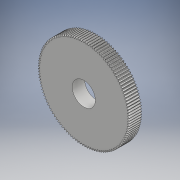
# Autodesk Inventor part: Колесо 1
Saved by Autodesk Inventor 2018.1 (Build 221171000, 171)
## iProperties
Created: 2018-06-08
Part Number: Колесо 1
Material: Типовые
Document SubType Name: Modeling
Designer: Dmitry
Density: 1 g/cm^3
Appearance: По умолчанию
Author: Dmitry
Autodesk Inventor part; units mm, degrees
ref_plane "YZ Plane" through (0, 0, 0) normal (1, 0, 0) x (0, 1, 0)
ref_plane "XZ Plane" through (0, 0, 0) normal (0, 1, 0) x (-1, 0, 0)
ref_plane "XY Plane" through (0, 0, 0) normal (0, 0, 1) x (1, 0, 0)
sketch "Эскиз1" plane through (0, 0, 0) normal (0, 0, 1) x (1, 0, 0)
  line L0 (31, 0) -> (122, 0)
  line L1 (122, 0) -> (122, 33.3333)
  line L2 (122, 33.3333) -> (31, 33.3333)
  line L3 (31, 33.3333) -> (31, 0)
  line L4 (0, -6.6667) -> (0, 40) projected
  constraints: 8 end point
revolve "Вращение1" add sketch "Эскиз1" angle 360 about axis through (0, -10, 0) along (0, 1, 0)
sketch "Эскиз2" plane through (0, 0, 0) normal (0, 1, 0) x (-1, 0, 0)
  line L0 (2.7475, 121.9691) -> (0.785, 117.7179)
  line L1 (-2.7475, 121.9691) -> (-0.785, 117.7179)
  arc A0 (2.7475, 121.9691) -> (-2.7475, 121.9691) centre (0, 0) ccw
  arc A1 (0.785, 117.7179) -> (-0.785, 117.7179) centre (0, 108.123) ccw
  constraints: 4 end point, 4 point on circle, 2 centre point
extrude "Выдавливание1" cut sketch "Эскиз2" along normal blind 33.3333
pattern_circular "Круговой массив1" count 120 over 360 about axis through (0, -10, 0) along (0, 1, 0) of "Выдавливание1"
